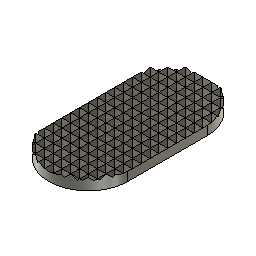
Anti-slip pad v2 (Autodesk Fusion 360 design; units mm, degrees)
Autodesk Fusion 360 part; units mm, degrees
sketch "Sketch1" plane through (0, 0, 0) normal (0, 0, 1) x (1, 0, 0)
  line L0 (-5, 10) -> (5, 10)
  line L1 (5, 10) -> (5, -10)
  line L2 (5, -10) -> (-5, -10)
  line L3 (-5, -10) -> (-5, 10)
  constraint horizontal L0
  constraint vertical L1
  constraint horizontal L2
  constraint vertical L3
extrude "Extrude1" add sketch "Sketch1" along normal blind 1
sketch "Sketch2" plane through (0, 0, 0) normal (1, 0, 0) x (0, 1, 0)
  line L0 (-10, 1) -> (-9.5, 1.5)
  line L1 (-9.5, 1.5) -> (-9, 1)
  line L2 (-9, 1) -> (-10, 1)
  line L3 (-8.5, 1.5) -> (-8, 1)
  line L4 (-9, 1) -> (-8.5, 1.5)
  line L5 (-8, 1) -> (-9, 1)
  line L6 (-7.5, 1.5) -> (-7, 1)
  line L7 (-8, 1) -> (-7.5, 1.5)
  line L8 (-7, 1) -> (-8, 1)
  line L9 (-6.5, 1.5) -> (-6, 1)
  line L10 (-7, 1) -> (-6.5, 1.5)
  line L11 (-6, 1) -> (-7, 1)
  line L12 (-5.5, 1.5) -> (-5, 1)
  line L13 (-6, 1) -> (-5.5, 1.5)
  line L14 (-5, 1) -> (-6, 1)
  line L15 (-4.5, 1.5) -> (-4, 1)
  line L16 (-5, 1) -> (-4.5, 1.5)
  line L17 (-4, 1) -> (-5, 1)
  line L18 (-3.5, 1.5) -> (-3, 1)
  line L19 (-4, 1) -> (-3.5, 1.5)
  line L20 (-3, 1) -> (-4, 1)
  line L21 (-2.5, 1.5) -> (-2, 1)
  line L22 (-3, 1) -> (-2.5, 1.5)
  line L23 (-2, 1) -> (-3, 1)
  line L24 (-1.5, 1.5) -> (-1, 1)
  line L25 (-2, 1) -> (-1.5, 1.5)
  line L26 (-1, 1) -> (-2, 1)
  line L27 (-0.5, 1.5) -> (0, 1)
  line L28 (-1, 1) -> (-0.5, 1.5)
  line L29 (0, 1) -> (-1, 1)
  line L30 (0.5, 1.5) -> (1, 1)
  line L31 (0, 1) -> (0.5, 1.5)
  line L32 (1, 1) -> (0, 1)
  line L33 (1.5, 1.5) -> (2, 1)
  line L34 (1, 1) -> (1.5, 1.5)
  line L35 (2, 1) -> (1, 1)
  line L36 (2.5, 1.5) -> (3, 1)
  line L37 (2, 1) -> (2.5, 1.5)
  line L38 (3, 1) -> (2, 1)
  line L39 (3.5, 1.5) -> (4, 1)
  line L40 (3, 1) -> (3.5, 1.5)
  line L41 (4, 1) -> (3, 1)
  line L42 (4.5, 1.5) -> (5, 1)
  line L43 (4, 1) -> (4.5, 1.5)
  line L44 (5, 1) -> (4, 1)
  line L45 (5.5, 1.5) -> (6, 1)
  line L46 (5, 1) -> (5.5, 1.5)
  line L47 (6, 1) -> (5, 1)
  line L48 (6.5, 1.5) -> (7, 1)
  line L49 (6, 1) -> (6.5, 1.5)
  line L50 (7, 1) -> (6, 1)
  line L51 (7.5, 1.5) -> (8, 1)
  line L52 (7, 1) -> (7.5, 1.5)
  line L53 (8, 1) -> (7, 1)
  line L54 (8.5, 1.5) -> (9, 1)
  line L55 (8, 1) -> (8.5, 1.5)
  line L56 (9, 1) -> (8, 1)
  line L57 (9.5, 1.5) -> (10, 1)
  line L58 (9, 1) -> (9.5, 1.5)
  line L59 (10, 1) -> (9, 1)
  dimension "d5" = 19
  dimension "d6" = 0
  constraint perpendicular L0 L1
  constraint horizontal L2
extrude "Extrude2" add sketch "Sketch2" along normal mid plane 10
sketch "Sketch3" plane through (0, 0, 0) normal (0, 1, 0) x (1, 0, 0)
  line L0 (5, -1) -> (4.5, -1.5)
  line L1 (4.5, -1.5) -> (5, -1.5)
  line L2 (5, -1.5) -> (5, -1)
  line L3 (-5, -1) -> (-5, -1.5)
  line L4 (-5, -1.5) -> (-4.5, -1.5)
  line L5 (-4.5, -1.5) -> (-5, -1)
  line L6 (4.5, -1.5) -> (4, -1)
  line L7 (4, -1) -> (3.5, -1.5)
  line L8 (3.5, -1.5) -> (4.5, -1.5)
  line L9 (3.5, -1.5) -> (3, -1)
  line L10 (2.5, -1.5) -> (3.5, -1.5)
  line L11 (3, -1) -> (2.5, -1.5)
  line L12 (2.5, -1.5) -> (2, -1)
  line L13 (1.5, -1.5) -> (2.5, -1.5)
  line L14 (2, -1) -> (1.5, -1.5)
  line L15 (1.5, -1.5) -> (1, -1)
  line L16 (0.5, -1.5) -> (1.5, -1.5)
  line L17 (1, -1) -> (0.5, -1.5)
  line L18 (0.5, -1.5) -> (0, -1)
  line L19 (-0.5, -1.5) -> (0.5, -1.5)
  line L20 (0, -1) -> (-0.5, -1.5)
  line L21 (-0.5, -1.5) -> (-1, -1)
  line L22 (-1.5, -1.5) -> (-0.5, -1.5)
  line L23 (-1, -1) -> (-1.5, -1.5)
  line L24 (-1.5, -1.5) -> (-2, -1)
  line L25 (-2.5, -1.5) -> (-1.5, -1.5)
  line L26 (-2, -1) -> (-2.5, -1.5)
  line L27 (-2.5, -1.5) -> (-3, -1)
  line L28 (-3.5, -1.5) -> (-2.5, -1.5)
  line L29 (-3, -1) -> (-3.5, -1.5)
  line L30 (-3.5, -1.5) -> (-4, -1)
  line L31 (-4.5, -1.5) -> (-3.5, -1.5)
  line L32 (-4, -1) -> (-4.5, -1.5)
  dimension "d11" = -8
  dimension "d12" = 0
  constraint horizontal L1
  constraint perpendicular L1 L2
  constraint perpendicular L1 L3
  constraint perpendicular L3 L4
  constraint perpendicular L0 L5
  constraint perpendicular L0 L6
  constraint perpendicular L6 L7
  constraint parallel L1 L8
extrude "Extrude3" cut sketch "Sketch3" along normal mid plane 20
sketch "Sketch4" plane through (0, 0, 0) normal (0, 0, 1) x (1, 0, 0)
  line L0 (5, -5.5) -> (5, 3.5)
  arc A0 (5, 3.5) -> (-4, 3.5) centre (0.5, 3.5) ccw
  line L1 (-4, 3.5) -> (-4, -5.5)
  arc A1 (-4, -5.5) -> (5, -5.5) centre (0.5, -5.5) ccw
  line L2 (0.5, -5.5) -> (0.5, 3.5) construction
  line L3 (5, 10) -> (5, -10)
  line L4 (5, -10) -> (-5, -10)
  dimension "d17" = 9
  dimension "d18" = 9
  constraint tangent L0 A0
  constraint tangent A0 L1
  constraint parallel L0 L1
  constraint tangent L1 A1
  constraint tangent L0 A1
  constraint vertical L2
  constraint coincident L0.start L3
  constraint tangent A1 L4
  measures "d17" distance of L0 L1
  measures "d18" distance of A1.centre A0.centre
extrude "Extrude4" cut sketch "Sketch4" along normal blind 2 contours L0 A0 L1 A1 L3 keep common part
